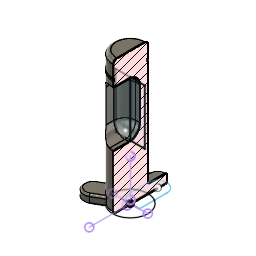
CandyDispenser (Autodesk Fusion 360 archive; units mm, degrees)
design "ガチャ_軸"
part number: 2025-12-10-21-28-01-673
Autodesk Fusion 360 part; units mm, degrees
sketch "スケッチ1" plane through (0, 0, 0) normal (0, 1, 0) x (1, 0, 0)
  circle A0 centre (0, 0) radius 9.6
  line L0 (-5, 0) -> (-5, 15)
  arc A1 (0, 20) -> (-5, 15) centre (0, 15) ccw
  line L1 (0, 20) -> (0, 0)
  line L2 (-5, 0) -> (0, 0)
  line L3 (0, -1.75) -> (0, -22.5)
  line L4 (5, 0) -> (5, 15)
  line L5 (5, 0) -> (0, 0)
  line L6 (0, 20) -> (0, 0)
  arc A2 (5, 15) -> (0, 20) centre (0, 15) ccw
  dimension "d1" = 19.2
  dimension "d2" = 15
  dimension "d4" = 5
  constraint coincident A0.centre L1.end
  constraint vertical L0
  constraint tangent L0 A1
  constraint vertical L1
  constraint perpendicular L1 L2
  constraint symmetric L0.start L3 L4.start
  constraint symmetric L0.end L3 L4.end
  constraint symmetric A1.start L3 L1.start
  constraint symmetric A1 L3 A2
  constraint symmetric A0.centre L3 L1.end
  measures "d1" diameter of A0
  measures "d2" vertical distance of A0.centre L0.end
  measures "d4" distance of L0.end A1.centre
extrude "押し出し1" add sketch "スケッチ1" along normal blind 73 contours A0 L0 L2 L4 L5 | A0 L1 L4 L5 L6 | A0 L0 L1 L2 L6 makes body 1
extrude "押し出し2" add sketch "スケッチ1" along normal blind 5 separate body contours A0 L1 L4 L5 L6 | A0 L1 L4 L6 A2 | A0 L0 L1 L2 L6 | A0 L0 A1 L1 L6 makes body 2
copy_body "ボディのコピーと貼り付け1" bodies 2 makes body 3
move_body "移動1" bodies 3 to x (-0.5, 0, -0.866025) y (0, 1, 0) z (0.866025, 0, -0.5) at (0, 0, 0)
copy_body "ボディのコピーと貼り付け2" bodies 3 makes body 4
move_body "移動2" bodies 4 to x (-0.5, 0, -0.866025) y (0, 1, 0) z (0.866025, 0, -0.5) at (0, 0, 0)
sketch "スケッチ2" plane through (0, 0, 0) normal (0, 0, 1) x (1, 0, 0)
  line L0 (0, 30) -> (8, 30)
  line L1 (8, 30) -> (8, 60)
  line L2 (8, 60) -> (0, 60)
  line L3 (0, 60) -> (0, 30)
  line L4 (9.6, 0) -> (-9.6, 0)
  line L5 (0, 1.75) -> (0, 22.5)
  line L6 (-8, 30) -> (-8, 60)
  line L7 (-8, 60) -> (0, 60)
  line L8 (0, 60) -> (0, 30)
  line L9 (0, 30) -> (-8, 30)
  dimension "d11" = 30
  dimension "d12" = 8
  dimension "d13" = 30
  constraint horizontal L0
  constraint vertical L1
  constraint horizontal L2
  constraint vertical L3
  constraint collinear L3 L5
  constraint symmetric L0.start L5 L3.end
  constraint symmetric L0.end L5 L6.start
  constraint symmetric L1.end L5 L6.end
  constraint symmetric L2.end L5 L3.start
  measures "d11" distance of L0 L4
  measures "d12" distance of L1.end L2.end
  measures "d13" distance of L0 L2
extrude "押し出し3" add sketch "スケッチ2" along normal blind 20 separate body makes body 5
move_body "移動3" bodies 5 to x (1, 0, 0) y (0, 1, 0) z (0, 0, 1) at (0, 0, -5)
combine "結合1" operation add target body 1 tool bodies 2 4 3
combine "結合2" operation cut target body 1 tool bodies 5
fillet "フィレット1" radius 6 8 edges at (8, 45, -5) (0, 60, -5) (8, 60, 0.1533) (-8, 60, 0.1533) (-8, 30, 0.1533) (0, 30, -5) (8, 30, 0.1533) (-8, 45, -5) on bodies 1
fillet "フィレット2" radius 2 1 edges at (-8.9503, 73, 3.4715) on bodies 1
fillet "フィレット3" radius 1 21 edges at (-12.5438, 5, 1.4687) (-17.3205, 5, 10) (-7.5438, 5, 10.1289) (7.5438, 5, 10.1289) (17.3205, 5, 10) (12.5438, 5, 1.4687) (5, 5, -11.5976) (0, 5, -20) (-5, 5, -11.5976) (7.5438, 0, 10.1289) (17.3205, 0, 10) (12.5438, 0, 1.4687) (5, 0, -11.5976) (0, 0, -20) (-5, 0, -11.5976) (-7.5438, 0, 10.1289) (-17.3205, 0, 10) (-12.5438, 0, 1.4687) (0, 0, 9.6) (8.3138, 0, -4.8) (-8.3138, 0, -4.8) on bodies 1
extrude "押し出し4" add sketch "スケッチ1" along normal blind 1.4 thin wall 0.4 on the right separate body open curves A0 makes body 6
move_body "移動4" bodies 6 to x (1, 0, 0) y (0, 1, 0) z (0, 0, 1) at (0, 63, 0)
combine "結合3" operation cut target body 1 tool bodies 6
fillet "フィレット5" radius 0.4 2 edges at (-8.5774, 64.4, -3.3269) (-8.5774, 63, 3.3269) on bodies 1
